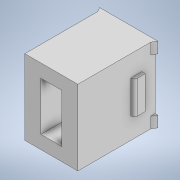
# Autodesk Inventor part: Porta Hall Sensor
Saved by Autodesk Inventor 2021 (Build 250183000, 183)
## iProperties
Created: 2021-08-29
Part Number: Porta Hall Sensor
Material: Genérico
Document SubType Name: Modeling
Designer: Diego.labarca
Density: 1 g/cm^3
Appearance: Valor por defecto
Author: Diego.labarca
Autodesk Inventor part; units mm, degrees
ref_plane "YZ Plane" through (0, 0, 0) normal (1, 0, 0) x (0, 1, 0)
ref_plane "XZ Plane" through (0, 0, 0) normal (0, 1, 0) x (-1, 0, 0)
ref_plane "XY Plane" through (0, 0, 0) normal (0, 0, 1) x (1, 0, 0)
sketch "Boceto1" plane through (0, 0, 0) normal (0, 0, 1) x (1, 0, 0)
  line L0 (-2.4, 3.4) -> (2.4, 3.4)
  line L1 (2.4, 3.4) -> (2.4, -3.4)
  line L2 (2.4, -3.4) -> (-2.4, -3.4)
  line L3 (-2.4, -3.4) -> (-2.4, 3.4)
  line L4 (-0.95, 2.2) -> (0.95, 2.2)
  line L5 (0.95, 2.2) -> (0.95, -2.2)
  line L6 (0.95, -2.2) -> (-0.95, -2.2)
  line L7 (-0.95, -2.2) -> (-0.95, 2.2)
  line L8 (0, -4.76) -> (0, 4.76) projected
  line L9 (-3.36, 0) -> (3.36, 0) projected
  dimension "d0" = 4.8
  dimension "d1" = 6.8
  dimension "d4" = 1.9
  dimension "d5" = 4.4
  constraints: 16 end point, 4 parallel, 2 horizontal, 2 perpendicular, 4 other
  measures "d0" distance of L1.end L2.end
  measures "d1" distance of L0.end L1.end
  measures "d4" distance of L5.end L6.end
  measures "d5" distance of L4.end L5.end
extrude "Extrusión1" add sketch "Boceto1" along normal blind 7 contours L0 L8 L4 L7 L9 L3 | L0 L1 L9 L5 L4 L8 | L9 L7 L6 L8 L2 L3 | L1 L2 L8 L6 L5 L9
sketch "Boceto2" plane through (2.4, -3.4, 0) normal (1, 0, 0) x (0, 0, -1)
  line L0 (-1.2, 4.8904) -> (-2.2, 4.8904)
  line L1 (-2.2, 4.8904) -> (-2.2, 1.9096)
  line L2 (-2.2, 1.9096) -> (-1.2, 1.9096)
  line L3 (-1.2, 1.9096) -> (-1.2, 4.8904)
  line L4 (1.4, 3.4) -> (-8.4, 3.4) projected
  line L5 (0, 0) -> (0, 6.8) projected
  point P0 (0, 3.4)
  dimension "d8" = 1.2
  dimension "d9" = 1
  constraints: 8 end point, 2 parallel, 1 horizontal, 1 perpendicular, 1 other
  measures "d8" distance between parallel lines of L3 L5
  measures "d9" distance of L0.start L0.end
extrude "Extrusión2" add sketch "Boceto2" along normal blind 0.3
sketch "Boceto3" plane through (-2.4, 3.4, 0) normal (0, 1, 0) x (1, 0, 0)
  line L0 (4.8, 0) -> (0, 0) projected
  line L1 (4.8, 0) -> (4.8, -0.4)
  line L2 (4.8, 0) -> (4.8, -7) projected
  line L3 (4.8, -0.4) -> (5.0309, 0)
  line L4 (5.0309, 0) -> (4.8, 0)
  point P0 (2.4, 0)
  dimension "d12" = 0.4
  dimension "d13" = 30
  constraints: 6 end point, 1 perpendicular, 1 point on line
  measures "d12" distance of L0.start L1.end
  measures "d13" angle of L3 L1
extrude "Extrusión3" add sketch "Boceto3" against normal blind 1
fillet "Empalme1" radius 0.3 1 edges at (2.7, 0, 2.2)
mirror "Simetría1" about plane through (0, 0, 0) normal (1, 0, 0) of "Extrusión2", "Empalme1"
mirror "Simetría2" about plane through (0, 0, 0) normal (1, 0, 0) of "Extrusión3"
mirror "Simetría3" about plane through (0, 0, 0) normal (0, 1, 0) of "Extrusión3", "Simetría2"
sketch "Boceto4" plane through (0, 0, 0) normal (0, 0, -1) x (-1, 0, 0)
  line L0 (-2.6309, 3.4) -> (2.6309, 3.4) projected
  line L1 (-2.6309, 3.4) -> (-2.6309, 2.4) projected
  line L2 (-2.4, 2.4) -> (-2.6309, 2.4) projected
  line L3 (-2.4, -2.4) -> (-2.4, 2.4) projected
  line L4 (-2.4, -2.4) -> (-2.6309, -2.4) projected
  line L5 (-2.6309, -3.4) -> (-2.6309, -2.4) projected
  line L6 (2.6309, -3.4) -> (-2.6309, -3.4) projected
  line L7 (2.6309, -3.4) -> (2.6309, -2.4) projected
  line L8 (2.4, -2.4) -> (2.6309, -2.4) projected
  line L9 (2.4, 2.4) -> (2.4, -2.4) projected
  line L10 (2.4, 2.4) -> (2.6309, 2.4) projected
  line L11 (2.6309, 3.4) -> (2.6309, 2.4) projected
  line L12 (0.95, 2.2) -> (-0.95, 2.2) projected
  line L13 (0.95, -2.2) -> (0.95, 2.2) projected
  line L14 (-0.95, -2.2) -> (0.95, -2.2) projected
  line L15 (-0.95, 2.2) -> (-0.95, -2.2) projected
  point P0 (0, 0)
extrude "Extrusión4" add sketch "Boceto4" against normal blind 0.6 contours L13 L14 L15 L12
